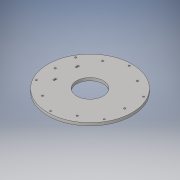
# Autodesk Inventor part: Turntable Top
Saved by Autodesk Inventor 2016 (Build 200138000, 138)
## iProperties
Created: 2016-04-25
Part Number: Turntable Top
Material: Generic
Document SubType Name: Modeling
Designer: rubenjm
Density: 1 g/cm^3
Appearance: Default
Author: rubenjm
Autodesk Inventor part; units mm, degrees
ref_plane "YZ Plane" through (0, 0, 0) normal (1, 0, 0) x (0, 1, 0)
ref_plane "XZ Plane" through (0, 0, 0) normal (0, 1, 0) x (-1, 0, 0)
ref_plane "XY Plane" through (0, 0, 0) normal (0, 0, 1) x (1, 0, 0)
sketch "Sketch1" plane through (0, 0, 0) normal (0, 1, 0) x (-1, 0, 0)
  circle A0 centre (0, 0) radius 190.5
  circle A1 centre (0, 0) radius 60.325
  dimension "d0" = 381
  dimension "d1" = 120.65
  constraints: 2 centre point, 2 coincident
  measures "d0" diameter of A0
  measures "d1" diameter of A1
extrude "Extrusion1" add sketch "Sketch1" along normal blind 12.7
sketch "Sketch2" plane through (0, 12.7, 0) normal (0, 1, 0) x (1, 0, 0)
  line L0 (-117.475, 63.5) -> (-111.125, 63.5)
  line L1 (-111.125, 63.5) -> (-111.125, 50.8)
  line L2 (-111.125, 50.8) -> (-117.475, 50.8)
  line L3 (-117.475, 50.8) -> (-117.475, 63.5)
  line L4 (-111.125, 50.8) -> (-111.125, -50.8) construction
  line L5 (-111.125, 50.8) -> (-212.725, 50.8) construction
  line L6 (-111.125, -50.8) -> (-117.475, -50.8)
  line L7 (-117.475, -50.8) -> (-117.475, -38.1)
  line L8 (-117.475, -38.1) -> (-111.125, -38.1)
  line L9 (-111.125, -38.1) -> (-111.125, -50.8)
  line L10 (-111.125, 0) -> (-60.325, 0) construction
  line L11 (-111.125, 0) -> (-60.325, 0) construction
  circle A0 centre (0, 0) radius 60.325 construction
  line L12 (0, 0) -> (-60.325, 0) construction
  dimension "d4" = 6.35
  dimension "d5" = 12.7
  dimension "d6" = 101.6
  dimension "d7" = 90
  dimension "d8" = 6.35
  dimension "d9" = 12.7
  dimension "d10" = 50.8
  dimension "d11" = 0
  constraints: 26 end point, 4 parallel, 3 horizontal, 2 equal length, 2 perpendicular, 1 coincident, 1 horizontal alignment, 1 midpoint, 2 other
  measures "d4" distance of L1.end L2.end
  measures "d5" distance of L0.end L1.end
  measures "d6" distance of L1.end L4.end
  measures "d7" angle of L5 L4
  measures "d8" distance of L7.end L8.end
  measures "d9" distance of L6.end L7.end
  measures "d10" distance of L10.start L10.end
  measures "d11" distance between parallel lines of L10 L11
extrude "Extrusion2" cut sketch "Sketch2" against normal through all
sketch "Sketch3" plane through (0, 12.7, 0) normal (0, 1, 0) x (1, 0, 0)
  circle A0 centre (0, 0) radius 157.48 construction
  circle A1 centre (-157.48, 0) radius 3.9687
  circle A2 centre (-78.74, -136.3817) radius 3.9687
  circle A3 centre (78.74, -136.3817) radius 3.9687
  circle A4 centre (157.48, 0) radius 3.9687
  circle A5 centre (78.74, 136.3817) radius 3.9687
  circle A6 centre (-78.74, 136.3817) radius 3.9687
  dimension "d16" = 314.96
  dimension "d17" = 7.9375
  dimension "d18" = 360
  constraints: 6 centre point, 1 coincident, 1 horizontal alignment, 15 other
  measures "d17" diameter of A1
extrude "Extrusion3" cut sketch "Sketch3" against normal through all
sketch "Sketch4" plane through (0, 12.7, 0) normal (0, 1, 0) x (1, 0, 0)
  line L0 (0, 0) -> (0, -177.8) construction
  line L1 (0, 0) -> (177.8, 0) construction
  circle A0 centre (0, -177.8) radius 3.81
  circle A1 centre (153.9793, -88.9) radius 3.81
  circle A2 centre (153.9793, 88.9) radius 3.81
  circle A3 centre (0, 177.8) radius 3.81
  circle A4 centre (-153.9793, 88.9) radius 3.81
  circle A5 centre (-153.9793, -88.9) radius 3.81
  dimension "d21" = 177.8
  dimension "d22" = 90
  dimension "d23" = 7.62
  dimension "d26" = 360
  constraints: 6 centre point, 4 end point, 1 coincident, 1 horizontal, 1 perpendicular, 1 vertical, 13 other
  measures "d21" distance of L0.start L0.end
  measures "d22" angle of L0 L1
  measures "d23" diameter of A0
extrude "Extrusion4" cut sketch "Sketch4" against normal through all
equation "\"d4\" = d8"
body "Solid1"
